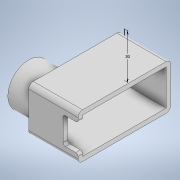
# Autodesk Inventor part: servo holder 1
Saved by Autodesk Inventor 2021 (Build 250183000, 183)
## iProperties
Created: 2021-01-31
Part Number: servo holder 1
Material: Generic
Document SubType Name: Modeling
Designer: josep
Density: 1 g/cm^3
Appearance: Default
Author: josep
Autodesk Inventor part; units mm, degrees
ref_plane "YZ Plane" through (0, 0, 0) normal (1, 0, 0) x (0, 1, 0)
ref_plane "XZ Plane" through (0, 0, 0) normal (0, 1, 0) x (-1, 0, 0)
ref_plane "XY Plane" through (0, 0, 0) normal (0, 0, 1) x (1, 0, 0)
sketch "Sketch1" plane through (0, 0, 0) normal (1, 0, 0) x (0, 1, 0)
  circle A0 centre (0, 0) radius 10
  circle A1 centre (0, 0) radius 14
  dimension "d0" = 20
  dimension "d1" = 28
  constraints: 2 centre point, 2 coincident
  measures "d0" diameter of A0
  measures "d1" diameter of A1
extrude "Extrusion1" add sketch "Sketch1" along normal blind 15
sketch "Sketch2" plane through (15, 0, 0) normal (1, 0, 0) x (0, 0, -1)
  point P0 (0, 0)
sketch "Sketch3" plane through (15, 0, 0) normal (1, 0, 0) x (0, 0, -1)
  circle A0 centre (0, 0) radius 10 projected
  line L0 (-12, 0) -> (-12, 12)
  line L1 (-12, 12) -> (46, 12)
  line L2 (46, 12) -> (46, -12)
  line L3 (46, -12) -> (-12, -12)
  line L4 (-12, -12) -> (-12, 0)
  line L5 (-15, 0) -> (-15, -12)
  line L6 (-15, 0) -> (-15, 12)
  line L7 (-12, 15) -> (46, 15)
  line L8 (49, 12) -> (49, -12)
  line L9 (46, -15) -> (-12, -15)
  arc A1 (49, 12) -> (46, 15) centre (46, 12) ccw
  arc A2 (46, -15) -> (49, -12) centre (46, -12) ccw
  arc A3 (-15, -12) -> (-12, -15) centre (-12, -12) ccw
  arc A4 (-12, 15) -> (-15, 12) centre (-12, 12) ccw
  constraints: 20 end point, 8 point on circle, 4 centre point, 4 perpendicular, 4 tangent, 3 point on line, 2 parallel, 1 vertical
extrude "Extrusion2" add sketch "Sketch3" along normal blind 33 contours L6 A4 L7 A1 L8 A2 L9 A3 L5
sketch "Sketch4" plane through (15, 0, 0) normal (1, 0, 0) x (0, 0, -1)
  line L0 (-12, -12) -> (-12, 12) projected
  line L1 (7.2111, 12) -> (46, 12) projected
  line L2 (-12, 12) -> (46, 12)
  line L3 (46, 12) -> (46, -12)
  line L4 (46, -12) -> (-12, -12) projected
  line L5 (46, -12) -> (-12, -12)
  line L6 (-12, 12) -> (46, 12) projected
  line L7 (-12, -12) -> (-12, 12)
  point P0 (0, 0)
  constraints: 8 end point, 2 collinear, 2 perpendicular
extrude "Extrusion3" add sketch "Sketch4" along normal blind 3
sketch "Sketch5" plane through (15, 0, 0) normal (-1, 0, 0) x (0, 0, 1)
  circle A0 centre (0, 0) radius 10
  constraints: 1 centre point, 1 coincident
extrude "Extrusion4" cut sketch "Sketch5" against normal blind 3
sketch "Sketch6" plane through (15, -12, -49) normal (0, 0, -1) x (-1, 0, 0)
  point P0 (15, 12)
sketch "Sketch7" plane through (15, -12, -49) normal (0, 0, -1) x (-1, 0, 0)
  line L0 (0, 0) -> (0, -3) projected
  line L1 (0, -3) -> (0, 27)
  point P0 (15, 12)
  dimension "d22" = 30
  constraints: 2 end point, 1 collinear
  measures "d22" distance of L0.end L1.end
sketch "Sketch8" plane through (15, -12, -49) normal (0, 0, -1) x (-1, 0, 0)
  point P0 (0, -3)
  point P1 (-3, 0)
sketch "Sketch9" plane through (15, -12, -49) normal (0, 0, -1) x (-1, 0, 0)
  line L0 (0, 27) -> (0, 24) projected
  line L1 (0, 27) -> (-64, 27)
  line L2 (-64, 27) -> (-64, -3)
  line L3 (0, -3) -> (-33, -3) projected
  line L4 (-64, -3) -> (0, -3)
  line L5 (0, -3) -> (0, 27)
  line L6 (0, 0) -> (0, 24) projected
  line L7 (-3, 24) -> (-3, 0) projected
  line L8 (-3, 0) -> (-3, 24)
  line L9 (0, 24) -> (-33, 24) projected
  line L10 (-3, 24) -> (-61, 24)
  line L11 (-61, 24) -> (-61, 0)
  line L12 (-61, 0) -> (-3, 0)
  line L13 (0, 0) -> (-33, 0) projected
  point P0 (15, 12)
  dimension "d27" = 64
  dimension "d28" = 30
  dimension "d29" = 58
  constraints: 16 end point, 3 perpendicular, 2 collinear, 1 horizontal, 1 parallel, 1 point on line
  measures "d27" distance of L0.start L1.end
  measures "d28" distance of L1.end L2.end
  measures "d29" distance of L8.end L10.end
extrude "Extrusion5" add sketch "Sketch9" along normal blind 30 contours L0 L9 L10 L11 L12 L13 L5 L3 L4 L2 L1 | L5 L13 L7 L9
sketch "Sketch10" plane through (48, 12, -49) normal (0, 0, -1) x (-1, 0, 0)
  line L0 (33, 3) -> (-31, 3) projected
  line L1 (33, 3) -> (33, 0) projected
  line L2 (-31, 3) -> (33, 3)
  line L3 (33, 3) -> (33, -27)
  line L4 (33, 0) -> (33, -24) projected
  line L5 (-31, 3) -> (-31, -27) projected
  line L6 (33, -27) -> (-31, -27)
  line L7 (-31, -27) -> (-31, 3)
  point P0 (48, -12)
  dimension "d32" = 30
  constraints: 8 end point, 2 collinear, 1 perpendicular
  measures "d32" distance of L0.start L3.end
extrude "Extrusion6" add sketch "Sketch10" against normal blind 5
fillet "Fillet1" radius 3 2 edges at (79, 15, -61.5) (79, -15, -61.5)
sketch "Sketch11" plane through (48, 12, -44) normal (0, 0, 1) x (1, 0, 0)
  line L0 (31, -24) -> (31, 0) projected
  line L1 (31, -12) -> (29, -12)
  line L2 (29, -12) -> (19, -12)
  circle A0 centre (19, -12) radius 10
  point P0 (-48, -12)
  dimension "d36" = 2
  dimension "d37" = 10
  constraints: 4 end point, 1 coincident, 1 horizontal, 1 horizontal alignment, 1 midpoint, 1 point on line, 2 other
  measures "d36" distance of L1.start L1.end
  measures "d37" distance of L1.end L2.end
extrude "Extrusion7" cut sketch "Sketch11" against normal blind 10.5
sketch "Sketch12" plane through (48, 12, -44) normal (0, 0, 1) x (1, 0, 0)
  arc A0 (28, -7.6411) -> (28, -16.3589) centre (19, -12) ccw projected
  circle A1 centre (19, -12) radius 10
  circle A2 centre (19, -12) radius 10 projected
  circle A3 centre (19, -12) radius 14
  point P0 (-48, -12)
  point P1 (28, -16.3589)
  dimension "d40" = 28
  constraints: 2 centre point, 2 coincident
  measures "d40" diameter of A3
extrude "Extrusion8" add sketch "Sketch12" along normal blind 15
sketch "Sketch13" plane through (15, -12, 15) normal (0, 0, 1) x (1, 0, 0)
  line L0 (33, 0) -> (3, 0) projected
  line L1 (0, -3) -> (33, -3) projected
  line L2 (30.6116, 0) -> (33.6116, 0) construction
  line L3 (33, 0) -> (33, 24) projected
  line L4 (33, 3) -> (23, 3)
  line L5 (23, 3) -> (23, 20.8588)
  line L6 (23, 20.8588) -> (33, 20.8588)
  point P0 (-15, 12)
  constraints: 8 end point, 3 perpendicular, 3 point on line, 1 horizontal
extrude "Extrusion9" cut sketch "Sketch13" against normal blind 21.75
sketch "Sketch14" plane through (79, -12, -79) normal (1, 0, 0) x (0, 0, -1)
  line L0 (-35, 24) -> (0, 24) projected
  line L1 (-3.7826, 24) -> (-0.7826, 24) construction
  line L2 (0, 0) -> (-35, 0) projected
  line L3 (-3.2489, 0) -> (-0.2489, 0) construction
  line L4 (0, 24) -> (0, 0) projected
  line L5 (0, 3) -> (-10, 3)
  line L6 (0, 3) -> (10, 3) construction
  line L7 (-10, 3) -> (-10, 21)
  line L8 (-10, 21) -> (0, 21)
  point P0 (-79, 12)
  dimension "d53" = 10
  dimension "d54" = 180
  constraints: 12 end point, 4 point on line, 3 horizontal, 3 perpendicular, 1 collinear
  measures "d53" distance of L5.start L5.end
  measures "d54" angle of L5 L6
extrude "Extrusion10" cut sketch "Sketch14" against normal blind 25.75
sketch "Sketch15" plane through (15, -12, -79) normal (0, 0, -1) x (-1, 0, 0)
  line L0 (8.5716, 47.3564) -> (-2.6139, -49.713)
  line L1 (-2.6139, -49.713) -> (-66.1269, -32.0991)
  line L2 (-66.1269, -32.0991) -> (-83.6498, 8.8041)
  line L3 (-83.6498, 8.8041) -> (-71.64, 52.1092)
  line L4 (-71.64, 52.1092) -> (-17.9136, 47.3564)
  arc A0 (-17.9136, 47.3564) -> (-17.9136, 47.3564) centre (-16.407, 64.3867) ccw
  line L5 (-17.9136, 47.3564) -> (8.5716, 47.3564)
  point P0 (15, 12)
  constraints: 12 end point, 2 point on circle, 1 centre point, 1 horizontal, 1 perpendicular, 1 point on line, 1 tangent
extrude "Extrusion11" cut sketch "Sketch15" against normal blind 30 contours L0 L1 L2 L3 L4 A0 L5 | A0 L5 picked at (-16.2394, 47.3367)
sketch "Sketch16" plane through (15, 15, 12) normal (0, 1, 0) x (1, 0, 0)
  line L0 (33, 56) -> (33, 0) projected
  line L1 (33, 35.3995) -> (33, 94.1554)
  line L2 (33, 94.1554) -> (79.7551, 84.127)
  line L3 (79.7551, 84.127) -> (69.5982, 12)
  line L4 (69.5982, 12) -> (67.3209, 12.3207)
  line L5 (67.3209, 12.3207) -> (33, 35.3995)
  point P0 (-15, 12)
  constraints: 10 end point, 1 point on line, 1 vertical
extrude "Extrusion12" cut sketch "Sketch16" against normal blind 77.25
sketch "Sketch18" plane through (48, -15, -49) normal (0, 0, -1) x (-1, 0, 0)
  point P0 (48, 15)
fillet "Fillet2" radius 3 2 edges at (31.5, 15, -49) (31.5, -15, -49)
sketch "Sketch19" plane through (48, -12, -49) normal (0, 0, -1) x (-1, 0, 0)
  line L0 (-10.3978, 34.6876) -> (55.1217, 36.4172)
  line L1 (55.1217, 36.4172) -> (42.8113, -19.5389)
  line L2 (42.8113, -19.5389) -> (-1.2413, -25.4397)
  arc A0 (-1.2413, -25.4397) -> (-3.1744, -22.4893) centre (-5.2865, -25.9815) ccw
  line L3 (-3.1744, -22.4893) -> (-13.3482, 5.1835)
  arc A1 (-13.3482, 5.1835) -> (-11.3134, 8.4392) centre (-14.4287, 8.1225) ccw
  line L4 (-11.3134, 8.4392) -> (-10.3978, 34.6876)
  point P0 (48, 12)
  constraints: 10 end point, 4 point on circle, 2 centre point, 2 point on line
extrude "Extrusion13" cut sketch "Sketch19" against normal blind 5
sketch "Sketch20" plane through (48, -12, -44) normal (0, 0, -1) x (-1, 0, 0)
  line L0 (0, 27) -> (0, 24) projected
  line L1 (0, 27) -> (33, 27)
  line L2 (33, 0) -> (33, -3) projected
  line L3 (33, 27) -> (33, -3)
  line L4 (33, -3) -> (0, -3) projected
  line L5 (33, -3) -> (0, -3)
  line L6 (0, -3) -> (0, 27)
  point P0 (48, 12)
  constraints: 8 end point, 3 perpendicular, 1 horizontal
extrude "Extrusion14" add sketch "Sketch20" along normal blind 3
fillet "Fillet3" radius 3 2 edges at (31.5, 15, -47) (31.5, -15, -47)
fillet "Fillet4" radius 1.5 4 edges at (48, 8.8588, 13.5) (38, 8.8588, 13.5) (38, -9, 13.5) (48, -9, 13.5)
body "Solid1"
